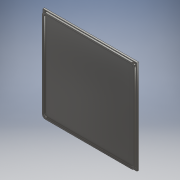
# Autodesk Inventor part: StackboxLid
Saved by Autodesk Inventor 2017 (Build 210142000, 142)
## iProperties
Created: 2017-10-10
Part Number: StackboxLid
Material: Generic
Document SubType Name: Modeling
Designer: Kathryn Rosie
Density: 1 g/cm^3
Appearance: Diamond Plate
Author: Kathryn Rosie
Autodesk Inventor part; units mm, degrees
ref_plane "YZ Plane" through (0, 0, 0) normal (1, 0, 0) x (0, 1, 0)
ref_plane "XZ Plane" through (0, 0, 0) normal (0, 1, 0) x (-1, 0, 0)
ref_plane "XY Plane" through (0, 0, 0) normal (0, 0, 1) x (1, 0, 0)
sketch "Sketch1" plane through (0, 0, 0) normal (1, 0, 0) x (0, 1, 0)
  line L0 (0, -300) -> (0.0001, 300)
  line L1 (0, 280) -> (0, -300) construction
  line L2 (-0.0001, -320) -> (0.0001, 300) construction
  line L3 (-9.9999, 300) -> (-9.9999, 295)
  line L4 (-9.9999, 295) -> (-19.9999, 295)
  line L5 (-10, -300) -> (-10, -295)
  line L6 (-10, -295) -> (-20, -295)
  line L7 (0, -300) -> (-10, -300)
  line L8 (-20, -295) -> (-19.9999, 295)
  line L9 (0.0001, 300) -> (-9.9999, 300)
  line L10 (0.0001, 0) -> (-19.9999, 0) construction
  point P0 (0, 0)
  dimension "d0" = 600
  dimension "d1" = 20
  dimension "d2" = 10
  dimension "d3" = 5
  dimension "d4" = 10
  dimension "d5" = 5
  dimension "d6" = 600
  dimension "d7" = 590
  dimension "d8" = 20
  constraints: 22 end point, 4 parallel, 3 point on line, 2 horizontal, 2 midpoint
  measures "d0" distance of L1.start L2.start
  measures "d1" distance of L0.start L2.start
  measures "d2" distance of L3.end L4.end
  measures "d3" distance of L3.start L3.end
  measures "d4" distance of L6.end L5.end
  measures "d5" distance of L5.end L5.start
  measures "d6" distance of L0.start L0.end
  measures "d7" distance of L6.end L4.end
  measures "d8" distance between parallel lines of L8 L0
extrude "Extrusion1" add sketch "Sketch1" along normal blind 600
sketch "Sketch2" plane through (0, -9.9999, 300) normal (0, 0, 1) x (1, 0, 0)
  line L0 (600, -10) -> (600, -10.0001) projected
  line L1 (600, -10.0001) -> (595, -10.0001)
  line L2 (595, -10.0001) -> (595, -0.0001)
  line L3 (595, -0.0001) -> (600, -0.0001)
  line L4 (600, -0.0001) -> (600, -10.0001)
  line L5 (5, 0) -> (-1, 0)
  line L6 (-1, 0) -> (-1, -11)
  line L7 (-1, -11) -> (5, -11)
  line L8 (5, -11) -> (5, 0)
  line L9 (0, 0) -> (0, -10) projected
  line L10 (0, 0) -> (600, 0) projected
  point P0 (0, 9.9999)
  dimension "d11" = 5
  dimension "d12" = 10
  dimension "d17" = 6
  dimension "d18" = 11
  dimension "d19" = 5
  constraints: 16 end point, 4 parallel, 2 horizontal, 2 perpendicular, 1 point on line
  measures "d11" distance of L2.end L3.end
  measures "d12" distance of L1.end L2.end
  measures "d17" distance of L5.start L5.end
  measures "d18" distance of L5.end L6.end
  measures "d19" distance between parallel lines of L9 L8
extrude "Extrusion2" cut sketch "Sketch2" against normal blind 600
shell "Shell1" thickness 10 removed faces 1 at (201.6667, -19.9999, 98.3333)
fillet "Fillet1" radius 20 4 edges at (5, -14.9999, 295) (595, -14.9999, 295) (595, -15, -295) (5, -15, -295)
fillet "Fillet2" radius 15 4 edges at (585, -15, -285) (585, -14.9999, 285) (15, -15, -285) (15, -14.9999, 285)
body "Solid1"
